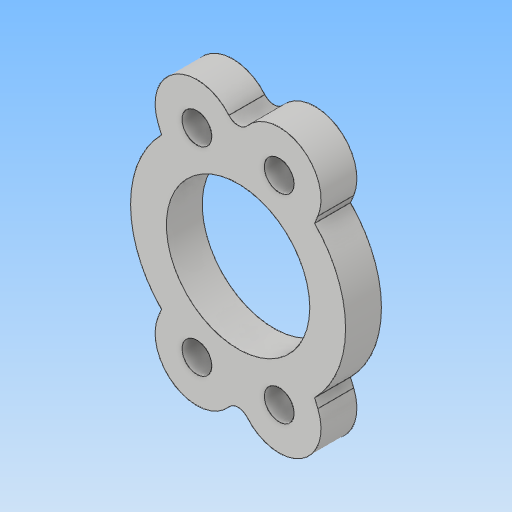
# Autodesk Inventor part: encoder_bearing_holder18_6mm_45
Saved by Autodesk Inventor 2020.2 (Build 242310000, 310)
## iProperties
Created: 2017-03-05
Part Number: encoder_bearing_holder18_6mm_45
Material: Allgemein
Document SubType Name: Modeling
Designer: paulg
Density: 1 g/cm^3
Appearance: Vorgabe
Author: paulg
Autodesk Inventor part; units mm, degrees
ref_plane "YZ Plane" through (0, 0, 0) normal (1, 0, 0) x (0, 1, 0)
ref_plane "XZ Plane" through (0, 0, 0) normal (0, 1, 0) x (-1, 0, 0)
ref_plane "XY Plane" through (0, 0, 0) normal (0, 0, 1) x (1, 0, 0)
sketch "Sketch1" plane through (0, 0, 0) normal (0, 0, 1) x (1, 0, 0)
  circle A0 centre (0, 0) radius 9
  line L0 (-3.4442, -8.3149) -> (3.4442, 8.3149) construction
  line L1 (-0.2106, -9.6543) -> (6.6777, 6.9755)
  line L2 (0.2106, 9.6543) -> (-6.6777, -6.9755)
  arc A1 (-6.6777, -6.9755) -> (-0.2106, -9.6543) centre (-3.4442, -8.3149) ccw
  arc A2 (6.6777, 6.9755) -> (0.2106, 9.6543) centre (3.4442, 8.3149) ccw
  line L3 (3.4442, -8.3149) -> (-3.4442, 8.3149) construction
  line L4 (6.6777, -6.9755) -> (-0.2106, 9.6543)
  line L5 (-6.6777, 6.9755) -> (0.2106, -9.6543)
  arc A3 (0.2106, -9.6543) -> (6.6777, -6.9755) centre (3.4442, -8.3149) ccw
  arc A4 (-0.2106, 9.6543) -> (-6.6777, 6.9755) centre (-3.4442, 8.3149) ccw
  line L6 (0, 0) -> (0, 9) construction
  dimension "d3" = 18
  dimension "d0" = 45
  dimension "d1" = 18
  dimension "d2" = 3.5
  constraints: 18 end point, 8 point on circle, 8 tangent, 4 centre point, 2 midpoint, 2 parallel, 1 coincident, 1 equal length, 1 equal radius, 1 vertical, 1 vertical alignment, 3 other
  measures "d0" angle of L0 L3
  measures "d1" distance of L3.start L3.end
  measures "d2" radius of A4
extrude "Extrusion1" add sketch "Sketch1" along normal blind 3
sketch "Sketch2" plane through (0, 0, 3) normal (0, 0, 1) x (1, 0, 0)
  arc A0 (-0.2106, 9.6543) -> (-6.6777, 6.9755) centre (-3.4442, 8.3149) ccw projected
  arc A1 (-6.6777, -6.9755) -> (-0.2106, -9.6543) centre (-3.4442, -8.3149) ccw projected
  arc A2 (0.2106, -9.6543) -> (6.6777, -6.9755) centre (3.4442, -8.3149) ccw projected
  arc A3 (6.4066, -6.321) -> (6.4066, 6.321) centre (0, 0) ccw projected
  arc A4 (6.6777, 6.9755) -> (0.2106, 9.6543) centre (3.4442, 8.3149) ccw projected
  circle A5 centre (-3.4442, 8.3149) radius 1.25
  circle A6 centre (3.4442, 8.3149) radius 1.25
  circle A7 centre (3.4442, -8.3149) radius 1.25
  circle A8 centre (-3.4442, -8.3149) radius 1.25
  circle A9 centre (0, 0) radius 6
  point P0 (0, 10.3491)
  point P1 (0, -10.3491)
  dimension "d6" = 2.5
  dimension "d7" = 12
  constraints: 5 centre point, 5 coincident, 3 equal radius, 4 other
  measures "d6" diameter of A5
  measures "d7" diameter of A9
extrude "Extrusion2" cut sketch "Sketch2" against normal through all
fillet "Fillet2" radius 1 2 edges at (0, -9.1459, 1.5) (0, 9.1459, 1.5)
sketch "Sketch3" plane through (0, 0, 3) normal (0, 0, 1) x (1, 0, 0)
  circle A0 centre (-3.4442, -8.3149) radius 1.25 projected
  circle A1 centre (3.4442, 8.3149) radius 1.25 projected
  circle A2 centre (-3.4442, 8.3149) radius 1.25 projected
  circle A3 centre (3.4442, -8.3149) radius 1.25 projected
  circle A4 centre (0, 0) radius 6 projected
  arc A5 (-6.4066, 6.321) -> (-6.4066, -6.321) centre (0, 0) ccw projected
  line L0 (-6.4066, -6.321) -> (-6.6777, -6.9755) projected
  arc A6 (-6.6777, -6.9755) -> (-0.7654, -10.5675) centre (-3.4442, -8.3149) ccw projected
  arc A7 (0.7654, -10.5675) -> (-0.7654, -10.5675) centre (0, -11.2111) ccw projected
  arc A8 (0.7654, -10.5675) -> (6.6777, -6.9755) centre (3.4442, -8.3149) ccw projected
  line L1 (6.6777, -6.9755) -> (6.4066, -6.321) projected
  arc A9 (6.4066, -6.321) -> (6.4066, 6.321) centre (0, 0) ccw projected
  line L2 (6.4066, 6.321) -> (6.6777, 6.9755) projected
  arc A10 (6.6777, 6.9755) -> (0.7654, 10.5675) centre (3.4442, 8.3149) ccw projected
  arc A11 (-0.7654, 10.5675) -> (0.7654, 10.5675) centre (0, 11.2111) ccw projected
  arc A12 (-0.7654, 10.5675) -> (-6.6777, 6.9755) centre (-3.4442, 8.3149) ccw projected
  line L3 (-6.6777, 6.9755) -> (-6.4066, 6.321) projected
  circle A13 centre (-3.4442, -8.3149) radius 3 construction
  dimension "d12" = 6
  constraints: 1 centre point, 1 coincident
  measures "d12" diameter of A13
body "Solid1"
